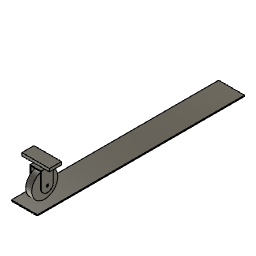
Testing Area_ (Autodesk Fusion 360 design; units mm, degrees)
Autodesk Fusion 360 part; units mm, degrees
note: some values were not read from the file. Set by a fixed rule: which sketch regions a step uses.
sketch "Sketch1" plane through (0, 0, 0) normal (0, 0, 1) x (1, 0, 0)
  line L0 (75, 600) -> (-75, 600)
  line L1 (-75, 600) -> (-75, -600)
  line L2 (-75, -600) -> (75, -600)
  line L3 (75, -600) -> (75, 600)
  line L4 (75, 600) -> (-75, -600) construction
  line L5 (-75, 600) -> (75, -600) construction
  dimension "d1" = 150
  dimension "d2" = 1200
  constraint horizontal L0
  constraint perpendicular L0 L1
  constraint parallel L0 L2
  constraint parallel L1 L3
  constraint coincident L4 origin
  constraint coincident L5 origin
  measures "d1" distance of L1.end L2.end
  measures "d2" distance of L0.end L1.end
extrude "Extrude1" add sketch "Sketch1" along normal blind 6 makes body 1
sketch "Sketch2" plane through (75, 0, 0) normal (1, 0, 0) x (0, 1, 0)
  line L0 (-600, 6) -> (-600, 0)
  line L1 (300, 6) -> (300, 156)
  line L2 (300, 156) -> (300, 258)
  line L3 (-600, 6) -> (-600, 258)
  line L4 (-600, 258) -> (300, 258)
  line L5 (-150, 258) -> (-150, 208)
  line L6 (300, 6) -> (-600, 6)
  line L7 (-150, 208) -> (-550, 208)
  line L8 (-150, 208) -> (250, 208)
  line L9 (250, 208) -> (250, 191)
  line L10 (250, 191) -> (-549.8941, 191)
  line L11 (-549.8941, 191) -> (-550, 208)
  point P0 (-150, 208)
  dimension "d5" = 150
  dimension "d6" = 102
  dimension "d7" = 252
  dimension "d47" = 50
  dimension "d48" = 900
  dimension "d49" = 400
  dimension "d50" = 400
  dimension "d51" = 17
  constraint parallel L1 L2
  constraint vertical L3
  constraint coincident L0.start L3.start
  constraint midpoint L4 L5.start
  constraint perpendicular L4 L5
  constraint coincident P0 L5.end
  constraint perpendicular L0 L6
  constraint perpendicular L5 L7
  constraint perpendicular L5 L8
  constraint vertical L9
  constraint perpendicular L9 L10
  constraint equal L4 L6
  measures "d5" distance of L1.start L1.end
  measures "d6" distance of L1.end L2.end
  measures "d7" distance of L0.start L3.end
  measures "d47" distance of L5.start P0
  measures "d48" distance of L1.start L0.start
  measures "d49" distance of P0 L7.end
  measures "d50" distance of P0 L8.end
  measures "d51" distance of L8.end L9.end
extrude "Extrude2" add sketch "Sketch2" along normal blind 5 separate body makes body 2
sketch "Sketch3" plane through (75, 0, 0) normal (-1, 0, 0) x (0, -1, 0)
  line L0 (-300, 258) -> (-300, 6)
  line L1 (600, 6) -> (600, 258)
  line L2 (600, 258) -> (-300, 258)
  line L3 (-300, 6) -> (600, 6)
  line L4 (-250, 208) -> (550, 208)
  line L5 (550, 208) -> (549.8941, 191)
  line L6 (549.8941, 191) -> (-250, 191)
  line L7 (-250, 191) -> (-250, 208)
sketch "Sketch4" plane through (75, 0, 0) normal (-1, 0, 0) x (0, -1, 0)
  line L0 (-300, 258) -> (-300, 6)
  line L1 (600, 6) -> (600, 258)
  line L2 (600, 258) -> (-300, 258)
  line L3 (499.7919, 201) -> (499.7919, 6)
  line L4 (499.7919, 6) -> (499.7919, 81)
  circle A0 centre (499.7919, 81) radius 75
  line L5 (-300, 6) -> (600, 6)
  line L6 (-250, 208) -> (550, 208)
  line L7 (550, 208) -> (549.8941, 191)
  line L8 (549.8941, 191) -> (-250, 191)
  line L9 (-250, 191) -> (-250, 208)
  dimension "d16" = 75
  constraint coincident L4.end A0.centre
  constraint coincident L3.end A0
  measures "d16" distance of L3.end L4.end
extrude "Extrude4" add sketch "Sketch4" along normal blind 92.5 separate body contours L3 L4 A0 | L3 L4 A0 makes body 3
move_face "OffsetFaces2" offset -57.5 1 faces at (75, -514.9596, 97.0923) on bodies 3
sketch "Sketch5" plane through (-17.5, 0, 0) normal (-1, 0, 0) x (0, -1, 0)
  circle A0 centre (499.7919, 81) radius 75
  circle A1 centre (499.7919, 81) radius 7.5
  dimension "d21" = 15
  constraint concentric A0 A1
  measures "d21" diameter of A1
extrude "Extrude5" cut sketch "Sketch5" against normal blind 35 contours A1 bodies 3
ref_plane "WorkPlane1" through (-27.5, -499.7919, 81) normal (-1, 0, 0) x (0, -1, 0)
sketch "Sketch6" plane through (-27.5, 0, 0) normal (-1, 0, 0) x (0, -1, 0)
  circle A0 centre (499.7919, 81) radius 7.5
  circle A1 centre (499.7919, 81) radius 35
  line L0 (499.7919, 81) -> (464.7919, 81)
  line L1 (499.7919, 81) -> (534.7919, 81)
  line L2 (534.7919, 81) -> (534.7919, 171)
  line L3 (464.7919, 81) -> (464.7919, 171)
  line L4 (464.7919, 171) -> (534.7919, 171)
  circle A2 centre (499.7919, 81) radius 75
  line L5 (499.7919, 171) -> (499.7919, 166)
  line L6 (499.7919, 166) -> (534.7919, 166)
  line L7 (499.7919, 166) -> (464.7919, 166)
  dimension "d26" = 70
  dimension "d27" = 90
  dimension "d28" = 90
  dimension "d31" = 5
  constraint concentric A0 A1
  constraint coincident A0.centre A1.centre
  constraint coincident A1 L0.end
  constraint horizontal L0
  constraint coincident A1 L1.end
  constraint parallel L0 L1
  constraint tangent A1 L2
  constraint perpendicular L0 L3
  constraint midpoint L4 L5.start
  constraint perpendicular L4 L5
  constraint coincident L2 L6.end
  constraint perpendicular L2 L6
  constraint coincident L3 L7.end
  constraint perpendicular L3 L7
  measures "d26" diameter of A1
  measures "d27" distance of L1.end L2.end
  measures "d28" distance of L0.end L3.end
  measures "d31" distance of L5.start L5.end
ref_plane "WorkPlane3" through (0, -499.7919, 81) normal (1, 0, 0) x (0, 1, 0)
extrude "Extrude6" add sketch "Sketch6" along normal blind 5 separate body contours A0 A1 L0 L1 | A0 A1 L0 L1 | A1 L2 L3 A2 | L2 L3 A2 L6 L7 | L2 L4 L5 L6 | L3 L4 L5 L7 picked at (524.2181, 137.4827) makes body 4
mirror "Mirror1" about plane through (0, -499.7919, 81) normal (1, 0, 0) of bodies 4 makes body 5
extrude "Extrude7" add sketch "Sketch6" against normal blind 55 contours L2 L4 L5 L6 | L3 L4 L5 L7 bodies 4 5
sketch "Sketch7" plane through (80, 0, 0) normal (1, 0, 0) x (0, 1, 0)
  line L0 (-550, 208) -> (250, 208)
  line L1 (250, 191) -> (-549.8941, 191)
  line L2 (-549.8941, 191) -> (-550, 208)
  line L3 (-550, 208) -> (-480.0014, 208.4361)
  line L4 (-480.0014, 208.4361) -> (-480.0014, 191)
  line L5 (-480.0014, 191) -> (-549.8941, 191)
  dimension "d54" = 70
  constraint coincident L0.start L2.end
  constraint perpendicular L2 L3
  constraint coincident L1 L4.end
  constraint perpendicular L1 L4
  constraint coincident L1.end L2.start
  measures "d54" distance of L0.start L3.end
extrude "Extrude8" add sketch "Sketch7" against normal blind 160 separate body contours L0 L1 L2 L4 L5 makes body 6
move_body "Align1" bodies 6 to x (1, 0, 0) y (0, 1, 0) z (0, 0, 1) at (0, 15.2094, 0)
sketch "Sketch11" plane through (80, 0, 0) normal (1, 0, 0) x (0, 1, 0)
  line L0 (-550, 208) -> (250, 208)
  line L1 (250, 208) -> (250, 191)
  line L2 (250, 191) -> (-549.8941, 191)
  line L3 (-549.8941, 191) -> (-550, 208)
  line L4 (300, 6) -> (300, 258)
  line L5 (300, 258) -> (-600, 258)
  line L6 (-600, 258) -> (-600, 6)
  line L7 (-600, 6) -> (300, 6)
hidden bodies 2
equation "d17 = 150.00 mm - 57.5 mm"
